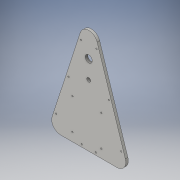
# Autodesk Inventor part: Nathan_LED_Speaker_Back
Saved by Autodesk Inventor 2016 (Build 200138000, 138)
## iProperties
Created: 2018-09-27
Part Number: Nathan_LED_Speaker_Back
Material: Generic
Document SubType Name: Modeling
Designer: Student
Density: 1 g/cm^3
Appearance: Default
Author: Student
Autodesk Inventor part; units mm, degrees
ref_plane "YZ Plane" through (0, 0, 0) normal (1, 0, 0) x (0, 1, 0)
ref_plane "XZ Plane" through (0, 0, 0) normal (0, 1, 0) x (-1, 0, 0)
sketch "Sketch1" plane through (0, 0, 0) normal (0, 0, 1) x (1, 0, 0)
  arc A0 (-2.400661, 17.597517) -> (12.7, -3.175) centre (12.7, 12.7) ccw
  arc A1 (114.3, -3.175) -> (129.400661, 17.597517) centre (114.3, 12.7) ccw
  line L0 (114.3, -3.175) -> (12.7, -3.175)
  line L1 (48.399339, 174.230681) -> (-2.400661, 17.597517)
  line L2 (129.400661, 17.597517) -> (78.600661, 174.230681)
  arc A2 (78.600661, 174.230681) -> (48.399339, 174.230681) centre (63.5, 169.333164) ccw
  arc A3 (75.580529, 173.251177) -> (51.419471, 173.251177) centre (63.5, 169.333164) ccw
  arc A4 (0.619471, 16.618013) -> (12.7, 0) centre (12.7, 12.7) ccw
  arc A5 (114.3, 0) -> (126.380529, 16.618013) centre (114.3, 12.7) ccw
  line L3 (12.7, 0) -> (114.3, 0)
  line L4 (0.619471, 16.618013) -> (51.419471, 173.251177)
  line L5 (75.580529, 173.251177) -> (126.380529, 16.618013)
  line L6 (0.619471, 16.618013) -> (3.753882, 26.282436)
  line L7 (3.753882, 26.282436) -> (4.961935, 25.890635)
  circle A6 centre (4.961935, 25.890635) radius 1.27
  line L8 (51.419471, 173.251177) -> (48.285061, 163.586755)
  line L9 (48.285061, 163.586755) -> (49.493113, 163.194953)
  circle A7 centre (49.493113, 163.194953) radius 1.27
  circle A8 centre (27.227524, 94.542794) radius 1.27
  line L10 (75.580529, 173.251177) -> (78.714939, 163.586755)
  line L11 (78.714939, 163.586755) -> (77.506886, 163.194953)
  circle A9 centre (77.506886, 163.194953) radius 1.27
  line L12 (126.380529, 16.618013) -> (123.246118, 26.282436)
  line L13 (123.246118, 26.282436) -> (122.038065, 25.890635)
  circle A10 centre (122.038065, 25.890635) radius 1.27
  circle A11 centre (99.772476, 94.542794) radius 1.27
  line L14 (63.5, 0) -> (63.5, 1.27) construction
  line L15 (63.5, 1.27) -> (76.2, 1.27) construction
  line L16 (63.5, 1.27) -> (50.8, 1.27) construction
  circle A12 centre (50.8, 1.27) radius 1.27
  circle A13 centre (76.2, 1.27) radius 1.27
  point P0 (0, 0)
  point P1 (0, 0)
  dimension "d50" = 2.54
  dimension "d53" = 2.54
  dimension "d39" = 31.75
  dimension "d40" = 31.75
  dimension "d41" = 25.4
  dimension "d42" = 25.4
  dimension "d43" = 25.4
  dimension "d44" = 10.16
  dimension "d45" = 10.16
  dimension "d46" = 1.27
  dimension "d47" = 1.27
  dimension "d48" = 10.16
  dimension "d49" = 10.16
  dimension "d51" = 2.54
  dimension "d52" = 2.54
  dimension "d91" = 12.7
  dimension "d92" = 12.7
  constraints: 34 end point, 12 point on circle, 10 centre point, 9 coincident, 6 tangent, 4 point on line, 2 perpendicular, 1 horizontal, 1 midpoint, 12 other
  measures "d39" diameter of A0
  measures "d40" diameter of A1
  measures "d41" diameter of A3
  measures "d42" diameter of A4
  measures "d43" diameter of A5
  measures "d44" distance of L4.start L7.start
  measures "d45" distance of L4.end L9.start
  measures "d46" distance of L9.start L9.end
  measures "d47" distance of L11.start L11.end
  measures "d48" distance of L5.end L12.end
  measures "d49" distance of L11.start L5.start
  measures "d51" diameter of A8
  measures "d52" diameter of A11
  measures "d91" distance of L14.end L15.end
  measures "d92" distance of L14.end L16.end
ref_plane "Work Plane1" through (0, 0, 4.572) normal (0, 0, 1) x (1, 0, 0)
sketch "Sketch2" plane through (0, 0, 4.572) normal (0, 0, 1) x (1, 0, 0)
  line L0 (12.7, -3.175) -> (114.3, -3.175)
  line L1 (34.171935, 12.065) -> (34.171935, 67.945) construction
  line L2 (34.171935, 67.945) -> (86.241935, 67.945) construction
  line L3 (86.241935, 67.945) -> (86.241935, 12.065) construction
  line L4 (86.241935, 12.065) -> (34.171935, 12.065) construction
  line L5 (34.171935, 12.065) -> (86.241935, 67.945) construction
  line L6 (34.171935, 67.945) -> (86.241935, 12.065) construction
  circle A0 centre (34.171935, 67.945) radius 1.27
  circle A1 centre (34.171935, 12.065) radius 1.27
  circle A2 centre (86.241935, 12.065) radius 1.27
  circle A3 centre (86.241935, 67.945) radius 1.27
  circle A4 centre (4.961935, 25.890635) radius 1.27
  circle A5 centre (63.5, 140.758164) radius 6.35
  arc A6 (78.600661, 174.230681) -> (48.399339, 174.230681) centre (63.5, 169.333164) ccw
  circle A7 centre (63.5, 108.090258) radius 3.429
  point P0 (0, 0)
  point P1 (60.206935, 40.005)
  dimension "d71" = 55.88
  dimension "d73" = 52.07
  dimension "d74" = 2.54
  dimension "d75" = 2.54
  dimension "d76" = 2.54
  dimension "d77" = 2.54
  dimension "d80" = 52.07
  dimension "d81" = 15.24
  dimension "d82" = 29.21
  dimension "d84" = 12.7
  dimension "d87" = 38.1
  dimension "d88" = 6.858
  constraints: 12 end point, 6 centre point, 4 coincident, 2 midpoint, 2 parallel, 1 perpendicular
  measures "d71" distance of L1.start L1.end
  measures "d73" distance of L1.end L2.end
  measures "d74" diameter of A0
  measures "d75" diameter of A1
  measures "d76" diameter of A2
  measures "d77" diameter of A3
  measures "d80" distance of A2.centre A1.centre
  measures "d81" distance between parallel lines of L4 L0
  measures "d82" distance from line of A4.centre L1
  measures "d84" diameter of A5
  measures "d88" diameter of A7
sketch "Sketch1 outline for Extrusion8" plane through (0, 0, 0) normal (0, 0, 1) x (1, 0, 0)
  arc A0 (78.600661, 174.230681) -> (48.399339, 174.230681) centre (63.5, 169.333164) ccw
  line L0 (129.400661, 17.597517) -> (78.600661, 174.230681)
  line L1 (48.399339, 174.230681) -> (-2.400661, 17.597517)
  arc A1 (114.3, -3.175) -> (129.400661, 17.597517) centre (114.3, 12.7) ccw
  arc A2 (-2.400661, 17.597517) -> (12.7, -3.175) centre (12.7, 12.7) ccw
  line L2 (12.7, -3.175) -> (114.3, -3.175)
  circle A3 centre (4.961935, 25.890635) radius 1.27
  circle A4 centre (50.8, 1.27) radius 1.27
  circle A5 centre (76.2, 1.27) radius 1.27
  circle A6 centre (122.038065, 25.890635) radius 1.27
  circle A7 centre (27.227524, 94.542794) radius 1.27
  circle A8 centre (49.493113, 163.194953) radius 1.27
  circle A9 centre (99.772476, 94.542794) radius 1.27
  circle A10 centre (77.506886, 163.194953) radius 1.27
extrude "Extrusion8" add sketch "Sketch1 outline for Extrusion8" along normal blind 4.572
extrude "Extrusion9" cut sketch "Sketch2" against normal blind 4.572 contours A0 | A1 | A2 | A3 | A5 | A7
body "Solid5"
